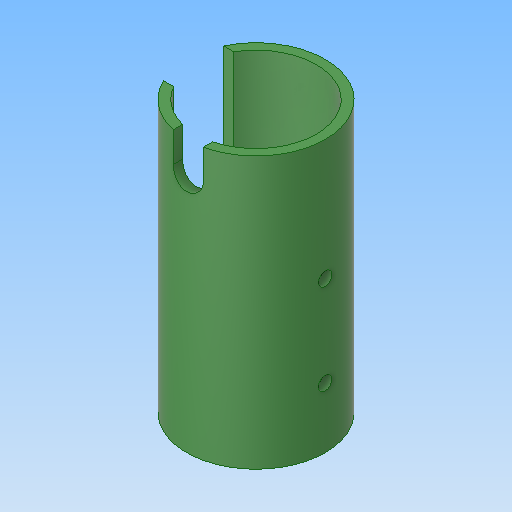
# Autodesk Inventor part: Pancake_PVC Pipe 2
Saved by Autodesk Inventor 2018.1 (Build 221171000, 171)
## iProperties
Created: 2019-02-11
Part Number: Pancake_PVC Pipe 2
Material: PVC-Piping
Document SubType Name: Modeling
Designer: James
Density: 1.4 g/cm^3
Appearance: Smooth - Dark Forest Green
Mass: 46.0258 g
Surface Area: 232.112 cm^2
Volume: 32.8755 cm^3
Author: James
Autodesk Inventor part; units mm, degrees
ref_plane "YZ Plane" through (0, 0, 0) normal (1, 0, 0) x (0, 1, 0)
ref_plane "XZ Plane" through (0, 0, 0) normal (0, 1, 0) x (-1, 0, 0)
ref_plane "XY Plane" through (0, 0, 0) normal (0, 0, 1) x (1, 0, 0)
sketch "Sketch1" plane through (0, 0, 0) normal (0, 1, 0) x (-1, 0, 0)
  circle A0 centre (0, 0) radius 23
  circle A1 centre (0, 0) radius 20
  dimension "d0" = 3
  dimension "d1" = 40
  constraints: 2 centre point, 2 coincident
  measures "d0" radial gap between concentric circles of A0 A1
  measures "d1" diameter of A1
extrude "Extrusion1" add sketch "Sketch1" along normal blind 90
sketch "Sketch2" plane through (0, 0, 0) normal (0, 0, 1) x (1, 0, 0)
  line L0 (-23, 100) -> (0, 100)
  line L1 (0, 100) -> (0, 40)
  line L2 (0, 40) -> (-23, 40)
  line L3 (-23, 40) -> (-23, 100)
  line L4 (23, 90) -> (-23, 90) projected
  line L5 (-23, 0) -> (23, 0) projected
  point P0 (0, 0)
  dimension "d4" = 60
  dimension "d34" = 40
  constraints: 8 end point, 2 parallel, 1 horizontal, 1 perpendicular, 1 vertical alignment
  measures "d4" distance of L2.end L0.start
  measures "d34" distance between parallel lines of L5 L2
extrude "Extrusion2" cut sketch "Sketch2" along normal mid plane 20
fillet "Fillet1" radius 5 2 edges at (-19.0164, 40, 10) (-19.0164, 40, -10)
sketch "Sketch3" plane through (0, 0, 0) normal (1, 0, 0) x (0, 1, 0)
  line L0 (-21, 0) -> (126, 0) projected
  line L1 (105, -5) -> (105, 5) projected
  line L2 (90, 20) -> (90, -20) projected
  line L3 (0, 23) -> (0, -23) projected
  point P0 (0, 0)
  point P1 (50, 0)
  point P2 (20, 0)
  dimension "d9" = 30
  dimension "d31" = 20
  constraints: 1 horizontal alignment, 1 point on line
  measures "d9" distance of point (20, 0) point (50, 0)
  measures "d31" distance from line of L3 point (20, 0)
hole "Hole1" at (0, 50, 0) at (0, 20, 0) direction (1, 0, 0) diameter 4.5 end through all clearance for "Socket Head Cap Screw" size "M4" standard "Ansi Metric M Profile"
sketch "Sketch4" plane through (0, 90, 0) normal (0, 1, 0) x (0, 0, -1)
  arc A0 (-10, 17.3205) -> (10, 17.3205) centre (0, 0) ccw projected
  arc A1 (-10, 20.7123) -> (10, 20.7123) centre (0, 0) ccw projected
  circle A2 centre (0, 0) radius 20 projected
  line L0 (10, 20.7123) -> (10, 17.3205) projected
  line L1 (-10, 17.3205) -> (-10, 20.7123) projected
  line L2 (-19.3649, -5) -> (-23, -5)
  line L3 (-23, -5) -> (-23, 5)
  line L4 (-23, 5) -> (-19.3649, 5)
  line L5 (-19.3649, 5) -> (-19.3649, -5)
  dimension "d32" = 10
  dimension "d33" = 5
  constraints: 8 end point, 2 parallel, 1 horizontal, 1 perpendicular, 1 tangent, 2 other
  measures "d32" distance of L2.end L3.end
  measures "d33" distance from line of L2 point (0, 0)
extrude "Extrusion3" cut sketch "Sketch4" against normal blind 15 contours L5 A0 | A0 L2 A1 L4 | A1 L3 L4 | L2 L3 A1
fillet "Fillet2" radius 5 2 edges at (5, 75, 20.9074) (-5, 75, 20.9074)
sketch "Sketch5" plane through (0, 0, 0) normal (0, 0, 1) x (1, 0, 0)
  line L0 (23, 90) -> (3, 90)
  line L1 (3, 90) -> (3, 60)
  line L2 (3, 60) -> (23, 60)
  line L3 (23, 60) -> (23, 90)
  line L4 (23, 0) -> (23, 90) projected
  line L5 (23, 90) -> (-20.7123, 90) projected
  point P0 (0, 0)
  point P1 (22.4499, 110)
  point P2 (22.4499, 110)
  dimension "d25" = 0
  dimension "d26" = 20
  dimension "d27" = 30
  constraints: 8 end point, 2 parallel, 1 coincident, 1 horizontal, 1 perpendicular, 1 other
  measures "d25" vertical extent of L0
  measures "d26" distance of L0.start L0.end
  measures "d27" distance between parallel lines of L2 L0
extrude "Extrusion4" [suppressed]
fillet "Fillet3" [suppressed]
equation "\"d33\" = 0.5 * d32"
body "Solid1"
